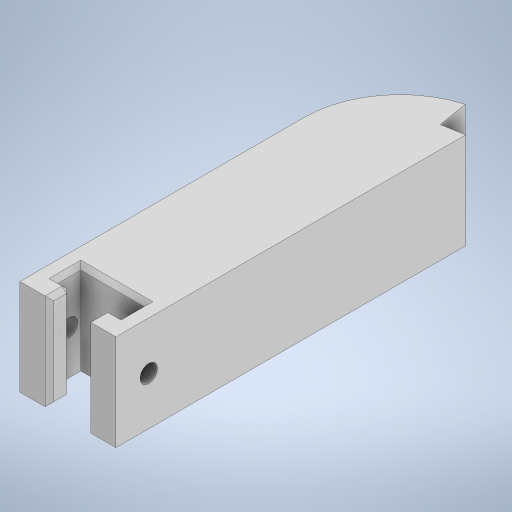
# Autodesk Inventor part: Gripper_V2_10deg
Saved by Autodesk Inventor 2024 (Build 280153000, 153)
## iProperties
Created: 2024-01-17
Part Number: Gripper_V2_10deg
Material: Generisch
Document SubType Name: Modeling
Designer: Zyc00pfg
Density: 1 g/cm^3
Appearance: Vorgabe
Author: Zyc00pfg
Autodesk Inventor part; units mm, degrees
ref_plane "YZ Plane" through (0, 0, 0) normal (1, 0, 0) x (0, 1, 0)
ref_plane "XZ Plane" through (0, 0, 0) normal (0, 1, 0) x (-1, 0, 0)
ref_plane "XY Plane" through (0, 0, 0) normal (0, 0, 1) x (1, 0, 0)
sketch "Skizze1" plane through (0, 0, 0) normal (0, 0, 1) x (1, 0, 0)
  line L0 (0, 0) -> (6.75, 0)
  line L1 (6.75, 0) -> (6.75, 4.9)
  line L2 (6.75, 4.9) -> (3.75, 4.9)
  line L3 (3.75, 4.9) -> (3.75, 10.2)
  line L4 (3.75, 10.2) -> (18.25, 10.2)
  line L5 (18.25, 10.2) -> (18.25, 4.9)
  line L6 (18.25, 4.9) -> (15.25, 4.9)
  line L7 (15.25, 4.9) -> (15.25, 0)
  line L8 (15.25, 0) -> (22, 0)
  line L9 (22, 0) -> (22, 80.2)
  line L10 (0, 0) -> (0, 65.0995)
  line L11 (22, 80.2) -> (22, 98.8308) construction
  line L12 (22, 80.2) -> (17.076, 79.3318)
  line L13 (17.076, 79.3318) -> (15.8604, 86.2254)
  arc A0 (22, 87.0995) -> (15.8604, 86.2254) centre (22, 65.0995) ccw construction
  arc A1 (15.8604, 86.2254) -> (0, 65.0995) centre (22, 65.0995) ccw
  dimension "d0" = 14.5
  dimension "d1" = 5.3
  dimension "d2" = 4.9
  dimension "d3" = 22
  dimension "d4" = 8.5
  dimension "d5" = 5
  dimension "d6" = 7
  dimension "d21" = 70
  dimension "d22" = 80
  constraints: 28 end point, 8 perpendicular, 5 point on line, 4 point on circle, 2 centre point, 2 collinear, 2 line through centre, 2 tangent, 2 vertical, 1 horizontal
  measures "d0" distance of L3.end L4.end
  measures "d1" distance of L4.end L5.end
  measures "d2" distance of L6.end L7.end
  measures "d3" distance between parallel lines of L10 L9
  measures "d4" distance between parallel lines of L7 L1
  measures "d5" distance of L9.end L12.end
  measures "d6" distance of L12.end L13.end
  measures "d21" distance from line of L9.end L4
  measures "d22" angle of L12 L9
extrude "Extrusion1" add sketch "Skizze1" along normal blind 22
sketch "Skizze2" plane through (22, 0, 0) normal (1, 0, 0) x (0, 0, -1)
  circle A0 centre (-11, 7.5) radius 2
  line L0 (0, 0) -> (-22, 0) projected
  line L1 (0, 0) -> (0, 80.2) projected
  point P0 (0, 65.2)
  dimension "d10" = 4
  dimension "d11" = 7.5
  dimension "d12" = 11
  constraints: 1 centre point
  measures "d10" diameter of A0
  measures "d11" distance from line of L0 A0.centre
  measures "d12" distance from line of L1 A0.centre
extrude "Extrusion2" cut sketch "Skizze2" against normal blind 22
chamfer "Fasen1" distance 1 angle 45 18 edges at (3.75, 7.55, 22) (11, 10.2, 22) (18.25, 7.55, 22) (16.75, 4.9, 22) (5.25, 4.9, 22) (6.75, 2.45, 22) (15.25, 2.45, 22) (18.25, 7.55, 0) (15.25, 2.45, 0) (16.75, 4.9, 0) (11, 10.2, 0) (3.75, 7.55, 0) (5.25, 4.9, 0) (6.75, 2.45, 0) (6.75, 4.9, 11) (15.25, 4.9, 11) (6.75, 0, 11) (15.25, 0, 11)
